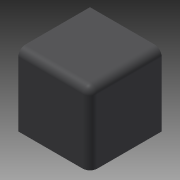
# Autodesk Inventor part: corner
Saved by Autodesk Inventor 2013 SP2 (Build 170200200, 200)
## iProperties
Created: 2018-09-21
Part Number: corner
Material: Generic
Document SubType Name: Modeling
Designer: alex
Density: 1 g/cm^3
Mass: 7.94984 g
Surface Area: 23.4535 cm^2
Volume: 7.94984 cm^3
Author: alex
Autodesk Inventor part; units mm, degrees
ref_plane "YZ Plane" through (0, 0, 0) normal (1, 0, 0) x (0, 1, 0)
ref_plane "XZ Plane" through (0, 0, 0) normal (0, 1, 0) x (-1, 0, 0)
ref_plane "XY Plane" through (0, 0, 0) normal (0, 0, 1) x (1, 0, 0)
sketch "Sketch1" plane through (0, 0, 0) normal (0, 0, 1) x (1, 0, 0)
  arc A0 (-0.804, -1.9351) -> (0.804, -1.9351) centre (0, 0) ccw projected
  arc A1 (-2.1249, -2.3045) -> (-0.804, -1.9351) centre (-1.5684, -1.748) ccw projected
  line L0 (-2.3045, -2.1249) -> (-2.1249, -2.3045) projected
  arc A2 (-1.9351, -0.804) -> (-2.3045, -2.1249) centre (-1.748, -1.5684) ccw projected
  arc A3 (-1.9351, 0.804) -> (-1.9351, -0.804) centre (0, 0) ccw projected
  arc A4 (-2.3045, 2.1249) -> (-1.9351, 0.804) centre (-1.748, 1.5684) ccw projected
  line L1 (-2.1249, 2.3045) -> (-2.3045, 2.1249) projected
  arc A5 (-0.804, 1.9351) -> (-2.1249, 2.3045) centre (-1.5684, 1.748) ccw projected
  arc A6 (0.804, 1.9351) -> (-0.804, 1.9351) centre (0, 0) ccw projected
  arc A7 (2.1249, 2.3045) -> (0.804, 1.9351) centre (1.5684, 1.748) ccw projected
  line L2 (2.3045, 2.1249) -> (2.1249, 2.3045) projected
  arc A8 (1.9351, 0.804) -> (2.3045, 2.1249) centre (1.748, 1.5684) ccw projected
  arc A9 (1.9351, -0.804) -> (1.9351, 0.804) centre (0, 0) ccw projected
  arc A10 (2.3045, -2.1249) -> (1.9351, -0.804) centre (1.748, -1.5684) ccw projected
  line L3 (2.1249, -2.3045) -> (2.3045, -2.1249) projected
  arc A11 (0.804, -1.9351) -> (2.1249, -2.3045) centre (1.5684, -1.748) ccw projected
  arc A12 (8.5, 5.487) -> (7.992, 5.995) centre (7.992, 5.487) ccw projected
  line L4 (8.5, 3.138) -> (8.5, 5.487) projected
  arc A13 (8.5, 3.138) -> (9.008, 2.63) centre (9.008, 3.138) ccw projected
  line L5 (9.492, 2.63) -> (9.008, 2.63) projected
  arc A14 (9.492, 2.63) -> (10, 3.138) centre (9.492, 3.138) ccw projected
  line L6 (10, 8.5) -> (10, 3.138) projected
  arc A15 (10, 8.5) -> (8.5, 10) centre (8.5, 8.5) ccw projected
  line L7 (3.138, 10) -> (8.5, 10) projected
  arc A16 (3.138, 10) -> (2.63, 9.492) centre (3.138, 9.492) ccw projected
  line L8 (2.63, 9.008) -> (2.63, 9.492) projected
  arc A17 (2.63, 9.008) -> (3.138, 8.5) centre (3.138, 9.008) ccw projected
  line L9 (5.487, 8.5) -> (3.138, 8.5) projected
  arc A18 (5.995, 7.992) -> (5.487, 8.5) centre (5.487, 7.992) ccw projected
  line L10 (5.995, 7.2661) -> (5.995, 7.992) projected
  arc A19 (5.8462, 6.9069) -> (5.995, 7.2661) centre (5.487, 7.2661) ccw projected
  line L11 (2.7431, 3.8038) -> (5.8462, 6.9069) projected
  arc A20 (2.3839, 3.655) -> (2.7431, 3.8038) centre (2.3839, 4.163) ccw projected
  line L12 (-2.3839, 3.655) -> (2.3839, 3.655) projected
  arc A21 (-2.7431, 3.8038) -> (-2.3839, 3.655) centre (-2.3839, 4.163) ccw projected
  line L13 (-5.8462, 6.9069) -> (-2.7431, 3.8038) projected
  arc A22 (-5.995, 7.2661) -> (-5.8462, 6.9069) centre (-5.487, 7.2661) ccw projected
  line L14 (-5.995, 7.992) -> (-5.995, 7.2661) projected
  arc A23 (-5.487, 8.5) -> (-5.995, 7.992) centre (-5.487, 7.992) ccw projected
  line L15 (-3.138, 8.5) -> (-5.487, 8.5) projected
  arc A24 (-3.138, 8.5) -> (-2.63, 9.008) centre (-3.138, 9.008) ccw projected
  line L16 (-2.63, 9.492) -> (-2.63, 9.008) projected
  arc A25 (-2.63, 9.492) -> (-3.138, 10) centre (-3.138, 9.492) ccw projected
  line L17 (-8.5, 10) -> (-3.138, 10) projected
  arc A26 (-8.5, 10) -> (-10, 8.5) centre (-8.5, 8.5) ccw projected
  line L18 (-10, 3.138) -> (-10, 8.5) projected
  arc A27 (-10, 3.138) -> (-9.492, 2.63) centre (-9.492, 3.138) ccw projected
  line L19 (-9.008, 2.63) -> (-9.492, 2.63) projected
  arc A28 (-9.008, 2.63) -> (-8.5, 3.138) centre (-9.008, 3.138) ccw projected
  line L20 (-8.5, 5.487) -> (-8.5, 3.138) projected
  arc A29 (-7.992, 5.995) -> (-8.5, 5.487) centre (-7.992, 5.487) ccw projected
  line L21 (-7.2661, 5.995) -> (-7.992, 5.995) projected
  arc A30 (-6.9069, 5.8462) -> (-7.2661, 5.995) centre (-7.2661, 5.487) ccw projected
  line L22 (-3.8038, 2.7431) -> (-6.9069, 5.8462) projected
  arc A31 (-3.655, 2.3839) -> (-3.8038, 2.7431) centre (-4.163, 2.3839) ccw projected
  line L23 (-3.655, -2.3839) -> (-3.655, 2.3839) projected
  arc A32 (-3.8038, -2.7431) -> (-3.655, -2.3839) centre (-4.163, -2.3839) ccw projected
  line L24 (-6.9069, -5.8462) -> (-3.8038, -2.7431) projected
  arc A33 (-7.2661, -5.995) -> (-6.9069, -5.8462) centre (-7.2661, -5.487) ccw projected
  line L25 (-7.992, -5.995) -> (-7.2661, -5.995) projected
  arc A34 (-8.5, -5.487) -> (-7.992, -5.995) centre (-7.992, -5.487) ccw projected
  line L26 (-8.5, -3.138) -> (-8.5, -5.487) projected
  arc A35 (-8.5, -3.138) -> (-9.008, -2.63) centre (-9.008, -3.138) ccw projected
  line L27 (-9.492, -2.63) -> (-9.008, -2.63) projected
  arc A36 (-9.492, -2.63) -> (-10, -3.138) centre (-9.492, -3.138) ccw projected
  line L28 (-10, -8.5) -> (-10, -3.138) projected
  arc A37 (-10, -8.5) -> (-8.5, -10) centre (-8.5, -8.5) ccw projected
  line L29 (-3.138, -10) -> (-8.5, -10) projected
  arc A38 (-3.138, -10) -> (-2.63, -9.492) centre (-3.138, -9.492) ccw projected
  line L30 (-2.63, -9.008) -> (-2.63, -9.492) projected
  arc A39 (-2.63, -9.008) -> (-3.138, -8.5) centre (-3.138, -9.008) ccw projected
  line L31 (-5.487, -8.5) -> (-3.138, -8.5) projected
  arc A40 (-5.995, -7.992) -> (-5.487, -8.5) centre (-5.487, -7.992) ccw projected
  line L32 (-5.995, -7.2661) -> (-5.995, -7.992) projected
  arc A41 (-5.8462, -6.9069) -> (-5.995, -7.2661) centre (-5.487, -7.2661) ccw projected
  line L33 (-2.7431, -3.8038) -> (-5.8462, -6.9069) projected
  arc A42 (-2.3839, -3.655) -> (-2.7431, -3.8038) centre (-2.3839, -4.163) ccw projected
  line L34 (2.3839, -3.655) -> (-2.3839, -3.655) projected
  arc A43 (2.7431, -3.8038) -> (2.3839, -3.655) centre (2.3839, -4.163) ccw projected
  line L35 (5.8462, -6.9069) -> (2.7431, -3.8038) projected
  arc A44 (5.995, -7.2661) -> (5.8462, -6.9069) centre (5.487, -7.2661) ccw projected
  line L36 (5.995, -7.992) -> (5.995, -7.2661) projected
  arc A45 (5.487, -8.5) -> (5.995, -7.992) centre (5.487, -7.992) ccw projected
  line L37 (3.138, -8.5) -> (5.487, -8.5) projected
  arc A46 (3.138, -8.5) -> (2.63, -9.008) centre (3.138, -9.008) ccw projected
  line L38 (2.63, -9.492) -> (2.63, -9.008) projected
  arc A47 (2.63, -9.492) -> (3.138, -10) centre (3.138, -9.492) ccw projected
  line L39 (8.5, -10) -> (3.138, -10) projected
  arc A48 (8.5, -10) -> (10, -8.5) centre (8.5, -8.5) ccw projected
  line L40 (10, -3.138) -> (10, -8.5) projected
  arc A49 (10, -3.138) -> (9.492, -2.63) centre (9.492, -3.138) ccw projected
  line L41 (9.008, -2.63) -> (9.492, -2.63) projected
  arc A50 (9.008, -2.63) -> (8.5, -3.138) centre (9.008, -3.138) ccw projected
  line L42 (8.5, -5.487) -> (8.5, -3.138) projected
  arc A51 (7.992, -5.995) -> (8.5, -5.487) centre (7.992, -5.487) ccw projected
  line L43 (7.2661, -5.995) -> (7.992, -5.995) projected
  arc A52 (6.9069, -5.8462) -> (7.2661, -5.995) centre (7.2661, -5.487) ccw projected
  line L44 (3.8038, -2.7431) -> (6.9069, -5.8462) projected
  arc A53 (3.655, -2.3839) -> (3.8038, -2.7431) centre (4.163, -2.3839) ccw projected
  line L45 (3.655, 2.3839) -> (3.655, -2.3839) projected
  arc A54 (3.8038, 2.7431) -> (3.655, 2.3839) centre (4.163, 2.3839) ccw projected
  line L46 (6.9069, 5.8462) -> (3.8038, 2.7431) projected
  arc A55 (7.2661, 5.995) -> (6.9069, 5.8462) centre (7.2661, 5.487) ccw projected
  line L47 (7.992, 5.995) -> (7.2661, 5.995) projected
  line L48 (10, -10) -> (-10, -10)
  line L49 (-10, -10) -> (-10, 10)
  line L50 (-10, 10) -> (10, 10)
  line L51 (10, 10) -> (10, -10)
  point P0 (0, 0)
  constraints: 8 end point, 2 parallel, 1 horizontal, 1 perpendicular
extrude "Extrusion1" add sketch "Sketch1" along normal blind 20 contours A1 L0 A2 A3 A4 L1 A5 A6 A7 L2 A8 A9 A10 L3 A11 A0 | L4 A13 L5 A14 L51 A49 L41 A50 L42 A51 L43 A52 L44 A53 L45 A54 L46 A55 L47 A12 | A12 L47 A55 L46 A54 L45 A53 L44 A52 L43 A51 L42 A50 L41 A49 L40 A48 L39 A47 L38 A46 L37 A45 L36 A44 L35 A43 L34 A42 L33 A41 L32 A40 L31 A39 L30 A38 L29 A37 L28 A36 L27 A35 L26 A34 L25 A33 L24 A32 L23 A31 L22 A30 L21 A29 L20 A28 L19 A27 L18 A26 L17 A25 L16 A24 L15 A23 L14 A22 L13 A21 L12 A20 L11 A19 L10 A18 L9 A17 L8 A16 L7 A15 L6 A14 L5 A13 L4 | A15 L50 L51 | L51 L48 A48 | A16 L8 A17 L9 A18 L10 A19 L11 A20 L12 A21 L13 A22 L14 A23 L15 A24 L16 A25 L50 | L48 A38 L30 A39 L31 A40 L32 A41 L33 A42 L34 A43 L35 A44 L36 A45 L37 A46 L38 A47 | A26 L49 L50 | L48 L49 A37 | A27 L19 A28 L20 A29 L21 A30 L22 A31 L23 A32 L24 A33 L25 A34 L26 A35 L27 A36 L49
fillet "Fillet1" radius 2 3 edges at (0, -10, 20) (10, -10, 10) (10, 0, 20)
body "Solid1"
